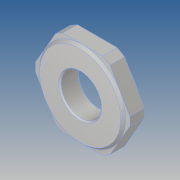
# Autodesk Inventor part: support_canon_ext
Saved by Autodesk Inventor 2019 (Build 230136000, 136)
## iProperties
Created: 2019-04-06
Part Number: support_canon_ext
Material: Aluminium 6061
Document SubType Name: Modeling
Designer: Theo
Density: 2.7 g/cm^3
Appearance: Aluminium - Plat
Author: Theo
Autodesk Inventor part; units mm, degrees
ref_plane "YZ Plane" through (0, 0, 0) normal (1, 0, 0) x (0, 1, 0)
ref_plane "XZ Plane" through (0, 0, 0) normal (0, 1, 0) x (-1, 0, 0)
sketch "Esquisse1" plane through (0, 0, 0) normal (0, 0, 1) x (1, 0, 0)
  circle A0 centre (0, 0) radius 17.5
  circle A1 centre (0, 0) radius 8.25
  dimension "d0" = 16.5
  dimension "d1" = 35
  constraints: 2 centre point, 2 coincident
  measures "d0" diameter of A1
  measures "d1" diameter of A0
extrude "Extrusion1" add sketch "Esquisse1" along normal blind 8
chamfer "Chanfrein1" distance 0.5 angle 45 2 edges at (-8.25, 0, 0) (-8.25, 0, 8)
chamfer "Chanfrein2" distance 1 angle 45 2 edges at (-17.5, 0, 8) (-17.5, 0, 0)
ref_plane "Plan de construction1" through (0, 0, 1) normal (0, 0, -1) x (-1, 0, 0)
sketch "Esquisse3" plane through (0, 0, 1) normal (0, 0, -1) x (-1, 0, 0)
  circle A0 centre (0, 0) radius 17.5 projected
  circle A1 centre (0, 0) radius 8.25 projected
  line L0 (10.1036, 17.5) -> (20.2073, 0)
  line L1 (20.2073, 0) -> (10.1036, -17.5)
  line L2 (10.1036, -17.5) -> (-10.1036, -17.5)
  line L3 (-10.1036, -17.5) -> (-20.2073, 0)
  line L4 (-20.2073, 0) -> (-10.1036, 17.5)
  line L5 (-10.1036, 17.5) -> (10.1036, 17.5)
  constraints: 12 end point, 1 coincident, 1 horizontal, 1 tangent, 13 other
extrude "Extrusion2" add sketch "Esquisse3" against normal blind 6 contours A0 L0 L1 | A0 L5 L0 | L1 L2 A0 | A0 L4 L5 | L2 L3 A0 | A0 L3 L4
chamfer "Chanfrein3" distance 2 angle 45 6 edges at (10.1036, 17.5, 4) (20.2073, 0, 4) (10.1036, -17.5, 4) (-10.1036, -17.5, 4) (-20.2073, 0, 4) (-10.1036, 17.5, 4)
sketch "Esquisse4" plane through (-8.1036, -17.5, 1) normal (0, -1, 0) x (1, 0, 0)
  line L0 (16.2073, 6) -> (16.2073, 0) projected
  point P0 (8.1036, -1)
  point P1 (8.1036, 3)
  point P2 (16.2073, 3)
  constraints: 1 horizontal alignment, 1 midpoint, 1 vertical alignment
hole "Perçage1" at (0, -17.5, 4) direction (0, 1, 0) diameter 3.242 depth 6 tip angle 118 thread size "M4x0.7" class "6H" standard "ISO Metric profile"
